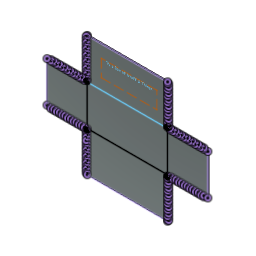
Shop_Box (Autodesk Fusion 360 design; units mm, degrees)
Autodesk Fusion 360 part; units mm, degrees
sketch "Sketch1" plane through (0, 0, 0) normal (0, 1, 0) x (1, 0, 0)
  line L0 (0, 0) -> (300, 0)
  line L1 (300, 0) -> (300, -150)
  line L2 (300, -150) -> (0, -150)
  line L3 (0, -150) -> (0, 0)
  line L4 (300, 0) -> (450, 0)
  line L5 (450, 0) -> (450, -150)
  line L6 (450, -150) -> (300, -150)
  line L7 (300, -150) -> (300, 0)
  line L8 (150, 0) -> (150, -150) construction
  line L9 (0, -75) -> (300, -75) construction
  line L10 (-150, -150) -> (0, -150)
  line L11 (0, 0) -> (0, -150)
  line L12 (-150, 0) -> (-150, -150)
  line L13 (0, 0) -> (-150, 0)
  line L14 (0, -150) -> (300, -150) construction
  line L15 (300, -150) -> (300, -300)
  line L16 (300, -300) -> (0, -300)
  line L17 (0, -300) -> (0, -150)
  line L18 (0, 150) -> (0, 0)
  line L19 (300, 0) -> (300, 150)
  line L20 (300, 150) -> (0, 150)
  line L21 (0, 0) -> (300, 0) construction
  line L22 (300, -150) -> (310.75, -150)
  line L23 (310.75, -150) -> (310.75, -154)
  line L24 (310.75, -154) -> (300, -154)
  line L25 (300, -154) -> (300, -150)
  line L26 (331.5, -150) -> (331.5, -154)
  line L27 (320.75, -150) -> (331.5, -150)
  line L28 (331.5, -154) -> (320.75, -154)
  line L29 (320.75, -154) -> (320.75, -150)
  line L30 (352.25, -150) -> (352.25, -154)
  line L31 (341.5, -150) -> (352.25, -150)
  line L32 (352.25, -154) -> (341.5, -154)
  line L33 (341.5, -154) -> (341.5, -150)
  line L34 (373, -150) -> (373, -154)
  line L35 (362.25, -150) -> (373, -150)
  line L36 (373, -154) -> (362.25, -154)
  line L37 (362.25, -154) -> (362.25, -150)
  line L38 (393.75, -150) -> (393.75, -154)
  line L39 (383, -150) -> (393.75, -150)
  line L40 (393.75, -154) -> (383, -154)
  line L41 (383, -154) -> (383, -150)
  line L42 (414.5, -150) -> (414.5, -154)
  line L43 (403.75, -150) -> (414.5, -150)
  line L44 (414.5, -154) -> (403.75, -154)
  line L45 (403.75, -154) -> (403.75, -150)
  line L46 (435.25, -150) -> (435.25, -154)
  line L47 (424.5, -150) -> (435.25, -150)
  line L48 (435.25, -154) -> (424.5, -154)
  line L49 (424.5, -154) -> (424.5, -150)
  line L50 (300, -150) -> (300, -160.25) construction
  line L51 (300, -160.25) -> (304, -160.25)
  line L52 (304, -160.25) -> (304, -171)
  line L53 (304, -171) -> (300, -171)
  line L54 (300, -171) -> (300, -160.25) construction
  line L55 (304, -181) -> (304, -191.75)
  line L56 (304, -191.75) -> (300, -191.75)
  line L57 (300, -181) -> (304, -181)
  line L58 (300, -191.75) -> (300, -181) construction
  line L59 (304, -201.75) -> (304, -212.5)
  line L60 (304, -212.5) -> (300, -212.5)
  line L61 (300, -201.75) -> (304, -201.75)
  line L62 (300, -212.5) -> (300, -201.75) construction
  line L63 (304, -222.5) -> (304, -233.25)
  line L64 (304, -233.25) -> (300, -233.25)
  line L65 (300, -222.5) -> (304, -222.5)
  line L66 (300, -233.25) -> (300, -222.5) construction
  line L67 (304, -243.25) -> (304, -254)
  line L68 (304, -254) -> (300, -254)
  line L69 (300, -243.25) -> (304, -243.25)
  line L70 (300, -254) -> (300, -243.25) construction
  line L71 (304, -264) -> (304, -274.75)
  line L72 (304, -274.75) -> (300, -274.75)
  line L73 (300, -264) -> (304, -264)
  line L74 (300, -274.75) -> (300, -264) construction
  line L75 (304, -284.75) -> (304, -295.5)
  line L76 (304, -295.5) -> (300, -295.5)
  line L77 (300, -284.75) -> (304, -284.75)
  line L78 (300, -295.5) -> (300, -284.75) construction
  line L79 (-4, -243.25) -> (-4, -254)
  line L80 (0, -243.25) -> (-4, -243.25)
  line L81 (0, -284.75) -> (-4, -284.75)
  line L82 (0, -160.25) -> (-4, -160.25)
  line L83 (0, -233.25) -> (0, -222.5) construction
  line L84 (0, -201.75) -> (-4, -201.75)
  line L85 (-4, -201.75) -> (-4, -212.5)
  line L86 (-4, -181) -> (-4, -191.75)
  line L87 (-4, -264) -> (-4, -274.75)
  line L88 (-4, -284.75) -> (-4, -295.5)
  line L89 (-4, -222.5) -> (-4, -233.25)
  line L90 (0, -191.75) -> (0, -181) construction
  line L91 (0, -212.5) -> (0, -201.75) construction
  line L92 (-4, -254) -> (0, -254)
  line L93 (-4, -233.25) -> (0, -233.25)
  line L94 (0, -254) -> (0, -243.25) construction
  line L95 (0, -295.5) -> (0, -284.75) construction
  line L96 (-4, -212.5) -> (0, -212.5)
  line L97 (0, -222.5) -> (-4, -222.5)
  line L98 (-4, -171) -> (0, -171)
  line L99 (-4, -274.75) -> (0, -274.75)
  line L100 (0, -171) -> (0, -160.25) construction
  line L101 (0, -274.75) -> (0, -264) construction
  line L102 (0, -264) -> (-4, -264)
  line L103 (0, -181) -> (-4, -181)
  line L104 (-4, -295.5) -> (0, -295.5)
  line L105 (-4, -191.75) -> (0, -191.75)
  line L106 (-4, -160.25) -> (-4, -171)
  line L107 (-31.5, -150) -> (-31.5, -154)
  line L108 (-83, -154) -> (-83, -150)
  line L109 (-103.75, -154) -> (-103.75, -150)
  line L110 (-83, -150) -> (-93.75, -150)
  line L111 (-124.5, -154) -> (-124.5, -150)
  line L112 (0, -150) -> (-10.75, -150)
  line L113 (-10.75, -150) -> (-10.75, -154)
  line L114 (-62.25, -154) -> (-62.25, -150)
  line L115 (-41.5, -150) -> (-52.25, -150)
  line L116 (-103.75, -150) -> (-114.5, -150)
  line L117 (-114.5, -150) -> (-114.5, -154)
  line L118 (-52.25, -150) -> (-52.25, -154)
  line L119 (-135.25, -150) -> (-135.25, -154)
  line L120 (-20.75, -150) -> (-31.5, -150)
  line L121 (-41.5, -154) -> (-41.5, -150)
  line L122 (-93.75, -150) -> (-93.75, -154)
  line L123 (-73, -150) -> (-73, -154)
  line L124 (-124.5, -150) -> (-135.25, -150)
  line L125 (-10.75, -154) -> (0, -154)
  line L126 (-150, -150) -> (0, -150)
  line L127 (-31.5, -154) -> (-20.75, -154)
  line L128 (0, -154) -> (0, -150)
  line L129 (-62.25, -150) -> (-73, -150)
  line L130 (-73, -154) -> (-62.25, -154)
  line L131 (-52.25, -154) -> (-41.5, -154)
  line L132 (-93.75, -154) -> (-83, -154)
  line L133 (-135.25, -154) -> (-124.5, -154)
  line L134 (-20.75, -154) -> (-20.75, -150)
  line L135 (-114.5, -154) -> (-103.75, -154)
  line L136 (-135.25, 4) -> (-124.5, 4)
  line L137 (0, 4) -> (0, 0)
  line L138 (-20.75, 0) -> (-31.5, 0)
  line L139 (-93.75, 0) -> (-93.75, 4)
  line L140 (-31.5, 4) -> (-20.75, 4)
  line L141 (-10.75, 4) -> (0, 4)
  line L142 (-83, 4) -> (-83, 0)
  line L143 (-73, 4) -> (-62.25, 4)
  line L144 (-135.25, 0) -> (-135.25, 4)
  line L145 (-83, 0) -> (-93.75, 0)
  line L146 (-124.5, 4) -> (-124.5, 0)
  line L147 (0, 0) -> (-10.75, 0)
  line L148 (-20.75, 4) -> (-20.75, 0)
  line L149 (-103.75, 4) -> (-103.75, 0)
  line L150 (-62.25, 0) -> (-73, 0)
  line L151 (-10.75, 0) -> (-10.75, 4)
  line L152 (-103.75, 0) -> (-114.5, 0)
  line L153 (-150, 0) -> (0, 0)
  line L154 (-41.5, 0) -> (-52.25, 0)
  line L155 (-41.5, 4) -> (-41.5, 0)
  line L156 (-73, 0) -> (-73, 4)
  line L157 (-62.25, 4) -> (-62.25, 0)
  line L158 (-31.5, 0) -> (-31.5, 4)
  line L159 (-150, 0) -> (0, 0)
  line L160 (-52.25, 0) -> (-52.25, 4)
  line L161 (-114.5, 0) -> (-114.5, 4)
  line L162 (-124.5, 0) -> (-135.25, 0)
  line L163 (-93.75, 4) -> (-83, 4)
  line L164 (-114.5, 4) -> (-103.75, 4)
  line L165 (-52.25, 4) -> (-41.5, 4)
  line L166 (424.5, 0) -> (435.25, 0)
  line L167 (435.25, 4) -> (424.5, 4)
  line L168 (435.25, 0) -> (435.25, 4)
  line L169 (320.75, 4) -> (320.75, 0)
  line L170 (331.5, 4) -> (320.75, 4)
  line L171 (414.5, 0) -> (414.5, 4)
  line L172 (373, 4) -> (362.25, 4)
  line L173 (403.75, 4) -> (403.75, 0)
  line L174 (414.5, 4) -> (403.75, 4)
  line L175 (383, 4) -> (383, 0)
  line L176 (352.25, 4) -> (341.5, 4)
  line L177 (393.75, 0) -> (393.75, 4)
  line L178 (331.5, 0) -> (331.5, 4)
  line L179 (450, 0) -> (300, 0)
  line L180 (300, 0) -> (310.75, 0)
  line L181 (310.75, 4) -> (300, 4)
  line L182 (450, 0) -> (300, 0)
  line L183 (341.5, 4) -> (341.5, 0)
  line L184 (300, 0) -> (450, 0)
  line L185 (310.75, 0) -> (310.75, 4)
  line L186 (362.25, 0) -> (373, 0)
  line L187 (300, 4) -> (300, 0)
  line L188 (362.25, 4) -> (362.25, 0)
  line L189 (341.5, 0) -> (352.25, 0)
  line L190 (373, 0) -> (373, 4)
  line L191 (320.75, 0) -> (331.5, 0)
  line L192 (393.75, 4) -> (383, 4)
  line L193 (403.75, 0) -> (414.5, 0)
  line L194 (383, 0) -> (393.75, 0)
  line L195 (352.25, 0) -> (352.25, 4)
  line L196 (424.5, 4) -> (424.5, 0)
  line L197 (300, 21) -> (300, 10.25) construction
  line L198 (300, 114) -> (304, 114)
  line L199 (300, 51.75) -> (304, 51.75)
  line L200 (304, 72.5) -> (304, 83.25)
  line L201 (304, 145.5) -> (300, 145.5)
  line L202 (300, 41.75) -> (300, 31) construction
  line L203 (304, 134.75) -> (304, 145.5)
  line L204 (300, 72.5) -> (304, 72.5)
  line L205 (300, 93.25) -> (304, 93.25)
  line L206 (304, 10.25) -> (304, 21)
  line L207 (300, 124.75) -> (300, 114) construction
  line L208 (304, 51.75) -> (304, 62.5)
  line L209 (304, 114) -> (304, 124.75)
  line L210 (304, 62.5) -> (300, 62.5)
  line L211 (300, 104) -> (300, 93.25) construction
  line L212 (300, 62.5) -> (300, 51.75) construction
  line L213 (300, 83.25) -> (300, 72.5) construction
  line L214 (304, 41.75) -> (300, 41.75)
  line L215 (300, 145.5) -> (300, 134.75) construction
  line L216 (304, 21) -> (300, 21)
  line L217 (300, 134.75) -> (304, 134.75)
  line L218 (304, 31) -> (304, 41.75)
  line L219 (304, 104) -> (300, 104)
  line L220 (300, 10.25) -> (304, 10.25)
  line L221 (304, 83.25) -> (300, 83.25)
  line L222 (304, 124.75) -> (300, 124.75)
  line L223 (300, 31) -> (304, 31)
  line L224 (304, 93.25) -> (304, 104)
  line L225 (0, 145.5) -> (0, 134.75) construction
  line L226 (-4, 62.5) -> (0, 62.5)
  line L227 (0, 124.75) -> (0, 114) construction
  line L228 (-4, 83.25) -> (0, 83.25)
  line L229 (0, 114) -> (-4, 114)
  line L230 (-4, 93.25) -> (-4, 104)
  line L231 (-4, 51.75) -> (-4, 62.5)
  line L232 (0, 51.75) -> (-4, 51.75)
  line L233 (-4, 104) -> (0, 104)
  line L234 (0, 21) -> (0, 10.25) construction
  line L235 (0, 83.25) -> (0, 72.5) construction
  line L236 (-4, 145.5) -> (0, 145.5)
  line L237 (0, 93.25) -> (-4, 93.25)
  line L238 (-4, 134.75) -> (-4, 145.5)
  line L239 (0, 104) -> (0, 93.25) construction
  line L240 (0, 31) -> (-4, 31)
  line L241 (-4, 41.75) -> (0, 41.75)
  line L242 (0, 10.25) -> (-4, 10.25)
  line L243 (-4, 114) -> (-4, 124.75)
  line L244 (0, 41.75) -> (0, 31) construction
  line L245 (-4, 124.75) -> (0, 124.75)
  line L246 (-4, 21) -> (0, 21)
  line L247 (-4, 10.25) -> (-4, 21)
  line L248 (0, 134.75) -> (-4, 134.75)
  line L249 (-4, 72.5) -> (-4, 83.25)
  line L250 (0, 62.5) -> (0, 51.75) construction
  line L251 (-4, 31) -> (-4, 41.75)
  line L252 (0, 72.5) -> (-4, 72.5)
  line L253 (0, -300) -> (300, -300) construction
  line L254 (60, -246.3912) -> (237.5858, -246.3912) construction
  line L255 (237.5858, -246.3912) -> (237.5858, -280) construction
  line L256 (237.5858, -280) -> (60, -280) construction
  line L257 (60, -280) -> (60, -246.3912) construction
  point P0 (320.75, -150)
  point P1 (320.75, -150)
  point P2 (341.5, -150)
  point P3 (341.5, -150)
  point P4 (362.25, -150)
  point P5 (362.25, -150)
  point P6 (383, -150)
  point P7 (383, -150)
  point P8 (403.75, -150)
  point P9 (403.75, -150)
  point P10 (424.5, -150)
  point P11 (424.5, -150)
  point P12 (0, -150)
  point P13 (-83, -150)
  point P14 (-124.5, -150)
  point P15 (-83, -150)
  point P16 (-20.75, -150)
  point P17 (-103.75, -150)
  point P18 (-62.25, -150)
  point P19 (-62.25, -150)
  point P20 (-20.75, -150)
  point P21 (-103.75, -150)
  point P22 (-41.5, -150)
  point P23 (-41.5, -150)
  point P24 (-124.5, -150)
  point P25 (-62.25, 0)
  point P26 (-103.75, 0)
  point P27 (-20.75, 0)
  point P28 (-83, 0)
  point P29 (-83, 0)
  point P30 (-20.75, 0)
  point P31 (-41.5, 0)
  point P32 (-41.5, 0)
  point P33 (-62.25, 0)
  point P34 (-124.5, 0)
  point P35 (-124.5, 0)
  point P36 (-103.75, 0)
  point P37 (383, 0)
  point P38 (320.75, 0)
  point P39 (320.75, 0)
  point P40 (424.5, 0)
  point P41 (383, 0)
  point P42 (362.25, 0)
  point P43 (424.5, 0)
  point P44 (403.75, 0)
  point P45 (341.5, 0)
  point P46 (341.5, 0)
  point P47 (362.25, 0)
  point P48 (403.75, 0)
  point P49 (300, 150)
  dimension "d7" = 300
  dimension "d8" = 150
  dimension "d9" = 150
  dimension "d10" = 150
  dimension "d11" = 300
  dimension "d12" = 150
  dimension "d15" = 10.75
  dimension "d16" = 4
  dimension "d19" = 0
  dimension "d20" = 0
  dimension "d23" = 20.75
  dimension "d24" = 0
  dimension "d25" = 10.25
  dimension "d26" = 4
  dimension "d27" = 10.75
  dimension "d30" = 20.75
  dimension "d31" = 0
  dimension "d33" = 300
  dimension "d39" = 600
  dimension "d40" = 150
  dimension "d43" = 10
  constraint horizontal L0
  constraint vertical L1
  constraint horizontal L2
  constraint vertical L3
  constraint coincident L0.start L3.end
  constraint horizontal L4
  constraint vertical L5
  constraint horizontal L6
  constraint vertical L7
  constraint midpoint L0 L8.start
  constraint midpoint L2 L8.end
  constraint midpoint L3 L9.start
  constraint midpoint L7 L9.end
  constraint symmetric L0.end L8 L0.start
  constraint symmetric L1.end L8 P12
  constraint symmetric L4.end L8 L12.start
  constraint symmetric L5.end L8 L10.start
  constraint horizontal L14
  constraint vertical L15
  constraint horizontal L16
  constraint vertical L17
  constraint symmetric L9 P12 L0.start
  constraint symmetric L9 L1.end L0.end
  constraint symmetric L9 L15.end P49
  constraint horizontal L22
  constraint vertical L23
  constraint horizontal L24
  constraint vertical L25
  constraint perpendicular L2 L50
  constraint horizontal L51
  constraint vertical L52
  constraint horizontal L53
  constraint vertical L54
  constraint symmetric L8 L50.end L82.start
  constraint symmetric L8 L51.end L82.end
  constraint symmetric L8 L52.end L98.start
  constraint symmetric L8 L53.end L98.end
  constraint symmetric L8 L55.start L86.start
  constraint symmetric L8 L55.end L86.end
  constraint symmetric L8 L56.end L90.start
  constraint symmetric L8 L57.start L90.end
  constraint symmetric L8 L59.start L84.end
  constraint symmetric L8 L59.end L85.end
  constraint symmetric L8 L60.end L91.start
  constraint symmetric L8 L61.start L84.start
  constraint symmetric L8 L63.start L89.start
  constraint symmetric L8 L63.end L89.end
  constraint symmetric L8 L64.end L83.start
  constraint symmetric L8 L65.start L83.end
  constraint symmetric L8 L67.start L79.start
  constraint symmetric L8 L67.end L79.end
  constraint symmetric L8 L68.end L92.end
  constraint symmetric L8 L69.start L80.start
  constraint symmetric L8 L71.start L87.start
  constraint symmetric L8 L71.end L87.end
  constraint symmetric L8 L72.end L99.end
  constraint symmetric L8 L73.start L101.end
  constraint symmetric L8 L75.start L81.end
  constraint symmetric L8 L75.end L88.end
  constraint symmetric L8 L76.end L95.start
  constraint symmetric L8 L77.start L81.start
  constraint symmetric L8 L1.end P12
  constraint symmetric L8 L22.end L112.end
  constraint symmetric L8 L23.end L113.end
  constraint symmetric L8 L24.end L125.end
  constraint symmetric L8 L28.end L127.end
  constraint symmetric L8 P1 P20
  constraint symmetric L8 L26.end L107.end
  constraint symmetric L8 L26.start L107.start
  constraint symmetric L8 L32.end L121.start
  constraint symmetric L8 P3 P23
  constraint symmetric L8 L30.end L118.end
  constraint symmetric L8 L30.start L115.end
  constraint symmetric L8 L36.end L114.start
  constraint symmetric L8 P5 P19
  constraint symmetric L8 L34.end L123.end
  constraint symmetric L8 L34.start L123.start
  constraint symmetric L8 L40.end L108.start
  constraint symmetric L8 P7 P15
  constraint symmetric L8 L38.end L122.end
  constraint symmetric L8 L38.start L110.end
  constraint symmetric L8 L44.end L109.start
  constraint symmetric L8 P9 P21
  constraint symmetric L8 L42.end L117.end
  constraint symmetric L8 L42.start L116.end
  constraint symmetric L8 L48.end L111.start
  constraint symmetric L8 P11 P24
  constraint symmetric L8 L46.end L119.end
  constraint symmetric L8 L46.start L119.start
  constraint symmetric P12 L9 L0.start
  constraint symmetric L9 L10.start L12.start
  constraint symmetric L9 L110.end L139.start
  constraint symmetric L9 L112.end L147.end
  constraint symmetric L9 L113.end L141.start
  constraint symmetric L9 L125.end L137.start
  constraint symmetric L9 P15 P29
  constraint symmetric L9 L119.end L136.start
  constraint symmetric L9 P24 P35
  constraint symmetric L9 L119.start L144.start
  constraint symmetric L9 L122.end L139.end
  constraint symmetric L9 L127.end L140.end
  constraint symmetric L9 P20 P30
  constraint symmetric L9 L109.start L149.start
  constraint symmetric L9 P21 P36
  constraint symmetric L9 L108.start L142.start
  constraint symmetric L9 L107.end L140.start
  constraint symmetric L9 L123.start L150.end
  constraint symmetric L9 P19 P33
  constraint symmetric L9 L117.end L161.end
  constraint symmetric L9 L123.end L143.start
  constraint symmetric L9 L114.start L143.end
  constraint symmetric L9 L107.start L138.end
  constraint symmetric L9 L115.end L154.end
  constraint symmetric L9 L121.start L155.start
  constraint symmetric L9 P23 P32
  constraint symmetric L9 L116.end L152.end
  constraint symmetric L9 L118.end L160.end
  constraint symmetric L9 L111.start L136.end
  constraint symmetric L8 L0.start L0.end
  constraint symmetric L8 L12.start L4.end
  constraint symmetric L8 L154.end L189.end
  constraint symmetric L8 L147.end L180.end
  constraint symmetric L8 L139.start L177.start
  constraint symmetric L8 P33 P47
  constraint symmetric L8 L136.start L167.start
  constraint symmetric L8 P29 P41
  constraint symmetric L8 P36 P48
  constraint symmetric L8 P30 P39
  constraint symmetric L8 L138.end L178.start
  constraint symmetric L8 L143.end L172.end
  constraint symmetric L8 L152.end L171.start
  constraint symmetric L8 L140.end L169.start
  constraint symmetric L8 L150.end L186.end
  constraint symmetric L8 L140.start L170.start
  constraint symmetric L8 L142.start L175.start
  constraint symmetric L8 L155.start L176.end
  constraint symmetric L8 P32 P46
  constraint symmetric L8 P35 P43
  constraint symmetric L8 L141.start L181.start
  constraint symmetric L8 L137.start L181.end
  constraint symmetric L8 L143.start L172.start
  constraint symmetric L8 L136.end L167.end
  constraint symmetric L8 L161.end L171.end
  constraint symmetric L8 L144.start L166.end
  constraint symmetric L8 L160.end L176.start
  constraint symmetric L8 L139.end L177.end
  constraint symmetric L8 L149.start L173.start
  constraint symmetric L9 L50.end L197.end
  constraint symmetric L9 L51.end L206.start
  constraint symmetric L9 L52.end L206.end
  constraint symmetric L9 L53.end L197.start
  constraint symmetric L9 L55.start L218.start
  constraint symmetric L9 L55.end L214.start
  constraint symmetric L9 L56.end L202.start
  constraint symmetric L9 L57.start L202.end
  constraint symmetric L9 L59.start L199.end
  constraint symmetric L9 L59.end L208.end
  constraint symmetric L9 L60.end L210.end
  constraint symmetric L9 L61.start L199.start
  constraint symmetric L9 L63.start L200.start
  constraint symmetric L9 L63.end L200.end
  constraint symmetric L9 L64.end L213.start
  constraint symmetric L9 L65.start L204.start
  constraint symmetric L9 L67.start L205.end
  constraint symmetric L9 L67.end L219.start
  constraint symmetric L9 L68.end L211.start
  constraint symmetric L9 L69.start L205.start
  constraint symmetric L9 L71.start L198.end
  constraint symmetric L9 L71.end L209.end
  constraint symmetric L9 L72.end L207.start
  constraint symmetric L9 L73.start L198.start
  constraint symmetric L9 L75.start L203.start
  constraint symmetric L9 L75.end L201.start
  constraint symmetric L9 L76.end L201.end
  constraint symmetric L9 L77.start L215.end
  constraint symmetric L9 L88.end L236.start
  constraint symmetric L9 L91.start L226.end
  constraint symmetric L9 L98.end L234.start
  constraint symmetric L9 L86.end L241.start
  constraint symmetric L9 L95.start L225.start
  constraint symmetric L9 L81.start L225.end
  constraint symmetric L9 L98.start L246.start
  constraint symmetric L9 L84.end L231.start
  constraint symmetric L9 L90.end L240.start
  constraint symmetric L9 L86.start L240.end
  constraint symmetric L9 L81.end L238.start
  constraint symmetric L9 L90.start L241.end
  constraint symmetric L9 L85.end L226.start
  constraint symmetric L9 L84.start L232.start
  constraint symmetric L9 L101.end L227.end
  constraint symmetric L9 L99.end L227.start
  constraint symmetric L9 L87.end L243.end
  constraint symmetric L9 L87.start L229.end
  constraint symmetric L9 L89.start L249.start
  constraint symmetric L9 L80.start L237.start
  constraint symmetric L9 L79.end L230.end
  constraint symmetric L9 L92.end L233.end
  constraint symmetric L9 L79.start L230.start
  constraint symmetric L9 L83.end L235.end
  constraint symmetric L9 L83.start L228.end
  constraint symmetric L9 L89.end L228.start
  constraint symmetric L9 L82.start L234.end
  constraint symmetric L9 L82.end L242.end
  constraint horizontal L253
  constraint perpendicular L18 L20
  measures "d7" distance of L0.start L0.end
  measures "d8" distance of L0.start P12
  measures "d9" distance of L0.end L4.end
  measures "d10" distance of L0.end L1.end
  measures "d11" distance of P12 L1.end
  measures "d12" distance of P12 L16.end
  measures "d15" distance of L1.end L22.end
  measures "d16" distance of L1.end L24.end
  measures "d25" distance of L1.end L50.end
  measures "d26" distance of L50.end L51.end
  measures "d27" distance of L50.end L53.end
  measures "d33" distance of L16.end L15.end
  measures "d39" distance of L5 L12
  measures "d40" distance of L0 L20
extrude "Extrude1" add sketch "Sketch1" along normal blind 4
sketch "Sketch2" plane through (0, 0, 0) normal (0, -1, 0) x (1, 0, 0)
  line L0 (0, -41.75) -> (0, -51.75)
  line L1 (0, -51.75) -> (-4, -51.75)
  line L2 (-4, -51.75) -> (-4, -62.5)
  line L3 (-4, -62.5) -> (0, -62.5)
  line L4 (0, -62.5) -> (0, -72.5)
  line L5 (0, -72.5) -> (-4, -72.5)
  line L6 (-4, -72.5) -> (-4, -83.25)
  line L7 (-4, -83.25) -> (0, -83.25)
  line L8 (0, -83.25) -> (0, -93.25)
  line L9 (0, -93.25) -> (-4, -93.25)
  line L10 (-4, -93.25) -> (-4, -104)
  line L11 (-4, -104) -> (0, -104)
  line L12 (0, -104) -> (0, -114)
  line L13 (0, -114) -> (-4, -114)
  line L14 (-4, -114) -> (-4, -124.75)
  line L15 (-4, -124.75) -> (0, -124.75)
  line L16 (0, -124.75) -> (0, -134.75)
  line L17 (0, -134.75) -> (-4, -134.75)
  line L18 (-4, -134.75) -> (-4, -145.5)
  line L19 (-4, -145.5) -> (0, -145.5)
  line L20 (0, -145.5) -> (0, -150)
  line L21 (0, -150) -> (300, -150)
  line L22 (300, -150) -> (300, -145.5)
  line L23 (300, -145.5) -> (304, -145.5)
  line L24 (304, -145.5) -> (304, -134.75)
  line L25 (304, -134.75) -> (300, -134.75)
  line L26 (300, -134.75) -> (300, -124.75)
  line L27 (300, -124.75) -> (304, -124.75)
  line L28 (304, -124.75) -> (304, -114)
  line L29 (304, -114) -> (300, -114)
  line L30 (300, -114) -> (300, -104)
  line L31 (300, -104) -> (304, -104)
  line L32 (304, -104) -> (304, -93.25)
  line L33 (304, -93.25) -> (300, -93.25)
  line L34 (300, -93.25) -> (300, -83.25)
  line L35 (300, -83.25) -> (304, -83.25)
  line L36 (304, -83.25) -> (304, -72.5)
  line L37 (304, -72.5) -> (300, -72.5)
  line L38 (300, -72.5) -> (300, -62.5)
  line L39 (300, -62.5) -> (304, -62.5)
  line L40 (304, -62.5) -> (304, -51.75)
  line L41 (304, -51.75) -> (300, -51.75)
  line L42 (300, -51.75) -> (300, -41.75)
  line L43 (300, -41.75) -> (304, -41.75)
  line L44 (304, -41.75) -> (304, -31)
  line L45 (304, -31) -> (300, -31)
  line L46 (300, -31) -> (300, -21)
  line L47 (300, -21) -> (304, -21)
  line L48 (304, -21) -> (304, -10.25)
  line L49 (304, -10.25) -> (300, -10.25)
  line L50 (300, -10.25) -> (300, -4)
  line L51 (300, -4) -> (310.75, -4)
  line L52 (310.75, -4) -> (310.75, 0)
  line L53 (310.75, 0) -> (320.75, 0)
  line L54 (320.75, 0) -> (320.75, -4)
  line L55 (320.75, -4) -> (331.5, -4)
  line L56 (331.5, -4) -> (331.5, 0)
  line L57 (331.5, 0) -> (341.5, 0)
  line L58 (341.5, 0) -> (341.5, -4)
  line L59 (341.5, -4) -> (352.25, -4)
  line L60 (352.25, -4) -> (352.25, 0)
  line L61 (352.25, 0) -> (362.25, 0)
  line L62 (362.25, 0) -> (362.25, -4)
  line L63 (362.25, -4) -> (373, -4)
  line L64 (373, -4) -> (373, 0)
  line L65 (373, 0) -> (383, 0)
  line L66 (383, 0) -> (383, -4)
  line L67 (383, -4) -> (393.75, -4)
  line L68 (393.75, -4) -> (393.75, 0)
  line L69 (393.75, 0) -> (403.75, 0)
  line L70 (403.75, 0) -> (403.75, -4)
  line L71 (403.75, -4) -> (414.5, -4)
  line L72 (414.5, -4) -> (414.5, 0)
  line L73 (414.5, 0) -> (424.5, 0)
  line L74 (424.5, 0) -> (424.5, -4)
  line L75 (424.5, -4) -> (435.25, -4)
  line L76 (435.25, -4) -> (435.25, 0)
  line L77 (435.25, 0) -> (450, 0)
  line L78 (450, 0) -> (450, 150)
  line L79 (450, 150) -> (435.25, 150)
  line L80 (435.25, 150) -> (435.25, 154)
  line L81 (435.25, 154) -> (424.5, 154)
  line L82 (424.5, 154) -> (424.5, 150)
  line L83 (424.5, 150) -> (414.5, 150)
  line L84 (414.5, 150) -> (414.5, 154)
  line L85 (414.5, 154) -> (403.75, 154)
  line L86 (403.75, 154) -> (403.75, 150)
  line L87 (403.75, 150) -> (393.75, 150)
  line L88 (393.75, 150) -> (393.75, 154)
  line L89 (393.75, 154) -> (383, 154)
  line L90 (383, 154) -> (383, 150)
  line L91 (383, 150) -> (373, 150)
  line L92 (373, 150) -> (373, 154)
  line L93 (373, 154) -> (362.25, 154)
  line L94 (362.25, 154) -> (362.25, 150)
  line L95 (362.25, 150) -> (352.25, 150)
  line L96 (352.25, 150) -> (352.25, 154)
  line L97 (352.25, 154) -> (341.5, 154)
  line L98 (341.5, 154) -> (341.5, 150)
  line L99 (341.5, 150) -> (331.5, 150)
  line L100 (331.5, 150) -> (331.5, 154)
  line L101 (331.5, 154) -> (320.75, 154)
  line L102 (320.75, 154) -> (320.75, 150)
  line L103 (320.75, 150) -> (310.75, 150)
  line L104 (310.75, 150) -> (310.75, 154)
  line L105 (310.75, 154) -> (300, 154)
  line L106 (300, 154) -> (300, 160.25)
  line L107 (300, 160.25) -> (304, 160.25)
  line L108 (304, 160.25) -> (304, 171)
  line L109 (304, 171) -> (300, 171)
  line L110 (300, 171) -> (300, 181)
  line L111 (300, 181) -> (304, 181)
  line L112 (304, 181) -> (304, 191.75)
  line L113 (304, 191.75) -> (300, 191.75)
  line L114 (300, 191.75) -> (300, 201.75)
  line L115 (300, 201.75) -> (304, 201.75)
  line L116 (304, 201.75) -> (304, 212.5)
  line L117 (304, 212.5) -> (300, 212.5)
  line L118 (300, 212.5) -> (300, 222.5)
  line L119 (300, 222.5) -> (304, 222.5)
  line L120 (304, 222.5) -> (304, 233.25)
  line L121 (304, 233.25) -> (300, 233.25)
  line L122 (300, 233.25) -> (300, 243.25)
  line L123 (300, 243.25) -> (304, 243.25)
  line L124 (304, 243.25) -> (304, 254)
  line L125 (304, 254) -> (300, 254)
  line L126 (300, 254) -> (300, 264)
  line L127 (300, 264) -> (304, 264)
  line L128 (304, 264) -> (304, 274.75)
  line L129 (304, 274.75) -> (300, 274.75)
  line L130 (300, 274.75) -> (300, 284.75)
  line L131 (300, 284.75) -> (304, 284.75)
  line L132 (304, 284.75) -> (304, 295.5)
  line L133 (304, 295.5) -> (300, 295.5)
  line L134 (300, 295.5) -> (300, 300)
  line L135 (300, 300) -> (0, 300)
  line L136 (0, 300) -> (0, 295.5)
  line L137 (0, 295.5) -> (-4, 295.5)
  line L138 (-4, 295.5) -> (-4, 284.75)
  line L139 (-4, 284.75) -> (0, 284.75)
  line L140 (0, 284.75) -> (0, 274.75)
  line L141 (0, 274.75) -> (-4, 274.75)
  line L142 (-4, 274.75) -> (-4, 264)
  line L143 (-4, 264) -> (0, 264)
  line L144 (0, 264) -> (0, 254)
  line L145 (0, 254) -> (-4, 254)
  line L146 (-4, 254) -> (-4, 243.25)
  line L147 (-4, 243.25) -> (0, 243.25)
  line L148 (0, 243.25) -> (0, 233.25)
  line L149 (0, 233.25) -> (-4, 233.25)
  line L150 (-4, 233.25) -> (-4, 222.5)
  line L151 (-4, 222.5) -> (0, 222.5)
  line L152 (0, 222.5) -> (0, 212.5)
  line L153 (0, 212.5) -> (-4, 212.5)
  line L154 (-4, 212.5) -> (-4, 201.75)
  line L155 (-4, 201.75) -> (0, 201.75)
  line L156 (0, 201.75) -> (0, 191.75)
  line L157 (0, 191.75) -> (-4, 191.75)
  line L158 (-4, 191.75) -> (-4, 181)
  line L159 (-4, 181) -> (0, 181)
  line L160 (0, 181) -> (0, 171)
  line L161 (0, 171) -> (-4, 171)
  line L162 (-4, 171) -> (-4, 160.25)
  line L163 (-4, 160.25) -> (0, 160.25)
  line L164 (0, 160.25) -> (0, 154)
  line L165 (0, 154) -> (-10.75, 154)
  line L166 (-10.75, 154) -> (-10.75, 150)
  line L167 (-10.75, 150) -> (-20.75, 150)
  line L168 (-20.75, 150) -> (-20.75, 154)
  line L169 (-20.75, 154) -> (-31.5, 154)
  line L170 (-31.5, 154) -> (-31.5, 150)
  line L171 (-31.5, 150) -> (-41.5, 150)
  line L172 (-41.5, 150) -> (-41.5, 154)
  line L173 (-41.5, 154) -> (-52.25, 154)
  line L174 (-52.25, 154) -> (-52.25, 150)
  line L175 (-52.25, 150) -> (-62.25, 150)
  line L176 (-62.25, 150) -> (-62.25, 154)
  line L177 (-62.25, 154) -> (-73, 154)
  line L178 (-73, 154) -> (-73, 150)
  line L179 (-73, 150) -> (-83, 150)
  line L180 (-83, 150) -> (-83, 154)
  line L181 (-83, 154) -> (-93.75, 154)
  line L182 (-93.75, 154) -> (-93.75, 150)
  line L183 (-93.75, 150) -> (-103.75, 150)
  line L184 (-103.75, 150) -> (-103.75, 154)
  line L185 (-103.75, 154) -> (-114.5, 154)
  line L186 (-114.5, 154) -> (-114.5, 150)
  line L187 (-114.5, 150) -> (-124.5, 150)
  line L188 (-124.5, 150) -> (-124.5, 154)
  line L189 (-124.5, 154) -> (-135.25, 154)
  line L190 (-135.25, 154) -> (-135.25, 150)
  line L191 (-135.25, 150) -> (-150, 150)
  line L192 (-150, 150) -> (-150, 0)
  line L193 (-150, 0) -> (-135.25, 0)
  line L194 (-135.25, 0) -> (-135.25, -4)
  line L195 (-135.25, -4) -> (-124.5, -4)
  line L196 (-124.5, -4) -> (-124.5, 0)
  line L197 (-124.5, 0) -> (-114.5, 0)
  line L198 (-114.5, 0) -> (-114.5, -4)
  line L199 (-114.5, -4) -> (-103.75, -4)
  line L200 (-103.75, -4) -> (-103.75, 0)
  line L201 (-103.75, 0) -> (-93.75, 0)
  line L202 (-93.75, 0) -> (-93.75, -4)
  line L203 (-93.75, -4) -> (-83, -4)
  line L204 (-83, -4) -> (-83, 0)
  line L205 (-83, 0) -> (-73, 0)
  line L206 (-73, 0) -> (-73, -4)
  line L207 (-73, -4) -> (-62.25, -4)
  line L208 (-62.25, -4) -> (-62.25, 0)
  line L209 (-62.25, 0) -> (-52.25, 0)
  line L210 (-52.25, 0) -> (-52.25, -4)
  line L211 (-52.25, -4) -> (-41.5, -4)
  line L212 (-41.5, -4) -> (-41.5, 0)
  line L213 (-41.5, 0) -> (-31.5, 0)
  line L214 (-31.5, 0) -> (-31.5, -4)
  line L215 (-31.5, -4) -> (-20.75, -4)
  line L216 (-20.75, -4) -> (-20.75, 0)
  line L217 (-20.75, 0) -> (-10.75, 0)
  line L218 (-10.75, 0) -> (-10.75, -4)
  line L219 (-10.75, -4) -> (0, -4)
  line L220 (0, -4) -> (0, -10.25)
  line L221 (0, -10.25) -> (-4, -10.25)
  line L222 (-4, -10.25) -> (-4, -21)
  line L223 (-4, -21) -> (0, -21)
  line L224 (0, -21) -> (0, -31)
  line L225 (0, -31) -> (-4, -31)
  line L226 (-4, -31) -> (-4, -41.75)
  line L227 (-4, -41.75) -> (0, -41.75)
  line L228 (0, 150) -> (0, 0)
  line L229 (0, 0) -> (300, 0)
  line L230 (300, 0) -> (300, 150)
  line L231 (300, 150) -> (0, 150)
  line L232 (0, 154) -> (0, 150)
  line L233 (0, -4) -> (0, 0)
  line L234 (300, 0) -> (300, -4)
  line L235 (300, 154) -> (300, 150)
  line L236 (52.8592, 190) -> (260, 190) construction
  line L237 (260, 190) -> (260, 252.9609) construction
  line L238 (260, 252.9609) -> (52.8592, 252.9609) construction
  line L239 (52.8592, 252.9609) -> (52.8592, 190) construction
  dimension "d44" = 10
  constraint coincident L228.end L229.start
  constraint perpendicular L219 L228
  constraint perpendicular L52 L229
  constraint perpendicular L103 L230
  constraint coincident L164.end L165.start
  constraint coincident L219.end L220.start
  constraint coincident L50.end L51.start
  constraint perpendicular L51 L234
  constraint coincident L105.end L106.start
equation "kerf = 0.25 mm"
equation "box_Length = 300 mm"
equation "box_Width = 200 mm"
equation "box_height = 150 mm"
equation "d7 = box_Length"
equation "d8 = box_height"
equation "d9 = box_height"
equation "d10 = box_height"
equation "d11 = box_Length"
equation "d12 = box_height"
equation "finger_Width = 10.5 mm"
equation "cardboard_Thickness = 4.00 mm"
equation "d15 = finger_Width + kerf"
equation "d16 = cardboard_Thickness"
equation "d23 = finger_Width * 2 - kerf"
equation "d25 = finger_Width - kerf"
equation "d26 = cardboard_Thickness"
equation "d27 = finger_Width + kerf"
equation "d30 = finger_Width * 2 - kerf"
equation "d33 = box_Length"
